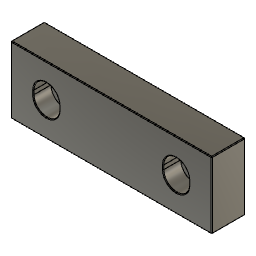
Soft Jaw (Autodesk Fusion 360 design; units mm, degrees)
Autodesk Fusion 360 part; units mm, degrees
sketch "Sketch1" plane through (0, 0, 0) normal (0, 1, 0) x (1, 0, 0)
  line L0 (76.2, 25.4) -> (-76.2, 25.4)
  line L1 (-76.2, 25.4) -> (-76.2, -25.4)
  line L2 (-76.2, -25.4) -> (76.2, -25.4)
  line L3 (76.2, -25.4) -> (76.2, 25.4)
  line L4 (76.2, 25.4) -> (-76.2, -25.4) construction
  line L5 (-76.2, 25.4) -> (76.2, -25.4) construction
  line L6 (-55.6895, 1.524) -> (-55.6895, -1.524)
  arc A0 (-55.6895, -1.524) -> (-42.7355, -1.524) centre (-49.2125, -1.524) ccw
  line L7 (-42.7355, -1.524) -> (-42.7355, 1.524)
  arc A1 (-42.7355, 1.524) -> (-55.6895, 1.524) centre (-49.2125, 1.524) ccw
  line L8 (-49.2125, 1.524) -> (-49.2125, -1.524) construction
  line L9 (0, 0) -> (0, -13.116) construction
  line L10 (-59.055, 1.524) -> (-59.055, -1.524)
  arc A2 (-59.055, -1.524) -> (-39.37, -1.524) centre (-49.2125, -1.524) ccw
  line L11 (-39.37, -1.524) -> (-39.37, 1.524)
  arc A3 (-39.37, 1.524) -> (-59.055, 1.524) centre (-49.2125, 1.524) ccw
  line L12 (-49.2125, 1.524) -> (-49.2125, -1.524) construction
  arc A4 (39.37, -1.524) -> (59.055, -1.524) centre (49.2125, -1.524) ccw
  line L13 (39.37, -1.524) -> (39.37, 1.524)
  arc A5 (59.055, 1.524) -> (39.37, 1.524) centre (49.2125, 1.524) ccw
  line L14 (59.055, 1.524) -> (59.055, -1.524)
  line L15 (55.6895, 1.524) -> (55.6895, -1.524)
  arc A6 (42.7355, -1.524) -> (55.6895, -1.524) centre (49.2125, -1.524) ccw
  line L16 (42.7355, -1.524) -> (42.7355, 1.524)
  arc A7 (55.6895, 1.524) -> (42.7355, 1.524) centre (49.2125, 1.524) ccw
  point P0 (-49.2125, 0)
  point P1 (-49.2125, 0)
  dimension "d1" = 152.4
  dimension "d2" = 50.8
  dimension "d3" = 49.2125
  dimension "d4" = 19.685
  dimension "d5" = 12.954
  dimension "d6" = 23.876
  dimension "d7" = 23.876
  constraint horizontal L0
  constraint perpendicular L0 L1
  constraint parallel L0 L2
  constraint parallel L1 L3
  constraint coincident L4 L9.start
  constraint coincident L5 L9.start
  constraint coincident L9.start origin
  constraint tangent L6 A0
  constraint tangent A0 L7
  constraint parallel L6 L7
  constraint tangent L7 A1
  constraint tangent L6 A1
  constraint perpendicular L2 L8
  constraint midpoint L8 P1
  constraint vertical L9
  constraint tangent L10 A2
  constraint tangent A2 L11
  constraint parallel L10 L11
  constraint tangent L11 A3
  constraint tangent L10 A3
  constraint coincident A0.centre L8.end
  constraint parallel L8 L12
  constraint coincident P1 P0
  constraint midpoint L12 P1
  constraint symmetric L6.start L9 L15.start
  constraint symmetric L6.end L9 L15.end
  constraint symmetric A0.end L9 A6.start
  constraint symmetric L7.end L9 L16.end
  constraint symmetric A0 L9 A6
  constraint symmetric A1 L9 A7
  constraint symmetric L9 L10.start A5.start
  constraint symmetric L9 L10.end A4.end
  constraint symmetric L9 A2.end A4.start
  constraint symmetric L9 L11.end L13.end
  constraint symmetric L9 A2 A4
  constraint symmetric L9 A3 A5
  measures "d1" distance of L1.end L2.end
  measures "d2" distance of L0.end L1.end
  measures "d3" distance of P1 L9
  measures "d4" distance of L10 L11
  measures "d5" distance of L6 L7
  measures "d6" distance of L2 A0.centre
  measures "d7" distance of L0 A1.centre
extrude "Extrude1" add sketch "Sketch1" along normal blind 25.4 contours L0 L1 L2 L3 | L6 A0 L7 A1 | L10 A2 L11 A3 | A4 L13 A5 L14 | L15 A6 L16 A7
extrude "Extrude2" cut sketch "Sketch1" along normal through all contours L6 A0 L7 A1 | L15 A6 L16 A7
extrude "Extrude3" cut sketch "Sketch1" along normal up to surface (13.335 mm away) contours L10 A2 L11 A3 | A4 L13 A5 L14
chamfer "Chamfer1" distance 0.508 angle 45 28 edges at (0, 0, 25.4) (76.2, 0, 0) (0, 0, -25.4) (-76.2, 0, 0) (-76.2, 12.7, 25.4) (-76.2, 25.4, 0) (-76.2, 12.7, -25.4) (0, 25.4, -25.4) (0, 25.4, 25.4) (76.2, 25.4, 0) (76.2, 12.7, 25.4) (76.2, 12.7, -25.4) (49.2125, 0, -11.3665) (39.37, 0, 0) (49.2125, 0, 11.3665) (59.055, 0, 0) (-39.37, 0, 0) (-49.2125, 0, -11.3665) (-59.055, 0, 0) (-49.2125, 0, 11.3665) (-55.6895, 25.4, 0) (-49.2125, 25.4, -8.001) (-42.7355, 25.4, 0) (-49.2125, 25.4, 8.001) (42.7355, 25.4, 0) (49.2125, 25.4, -8.001) (55.6895, 25.4, 0) (49.2125, 25.4, 8.001)
equation "d7 = d6"
named bodies: "SoftJaw"
